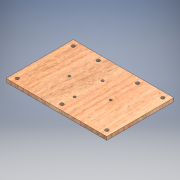
# Autodesk Inventor part: top
Saved by Autodesk Inventor 2018 (Build 220112000, 112)
## iProperties
Created: 2019-06-17
Part Number: top
Material: Generic
Document SubType Name: Modeling
Designer: ZEUSLAP
Density: 1 g/cm^3
Appearance: Default
Author: ZEUSLAP
Autodesk Inventor part; units mm, degrees
ref_plane "YZ Plane" through (0, 0, 0) normal (1, 0, 0) x (0, 1, 0)
ref_plane "XZ Plane" through (0, 0, 0) normal (0, 1, 0) x (-1, 0, 0)
ref_plane "XY Plane" through (0, 0, 0) normal (0, 0, 1) x (1, 0, 0)
sketch "Sketch1" plane through (0, 0, 0) normal (0, 0, 1) x (1, 0, 0)
  line L0 (-70, 40) -> (70, 40) construction
  line L1 (70, 40) -> (70, -40) construction
  line L2 (70, -40) -> (-70, -40) construction
  line L3 (-70, -40) -> (-70, 40) construction
  line L4 (90, 60) -> (-90, 60)
  line L5 (-90, 60) -> (-90, -60)
  line L6 (-90, -60) -> (90, -60)
  line L7 (90, -60) -> (90, 60)
  circle A0 centre (-80, -50) radius 3
  circle A1 centre (80, 50) radius 3
  circle A2 centre (0, -50) radius 3
  circle A3 centre (80, -50) radius 3
  circle A4 centre (-80, 50) radius 3
  line L8 (0, 60) -> (0, -60) construction
  line L9 (-90, 0) -> (90, 0) construction
  circle A5 centre (-35, 50) radius 3
  circle A6 centre (35, 50) radius 3
  circle A7 centre (0, 22.5) radius 2.15
  circle A8 centre (0, -27.5) radius 2.15
  circle A9 centre (37, 0) radius 2.15
  circle A10 centre (-37, 0) radius 2.15
  point P0 (0, 0)
  point P1 (-70, 0)
  point P2 (0, 40)
  point P3 (0, 0)
  dimension "d0" = 140
  dimension "d1" = 80
  dimension "d2" = 20
  dimension "d3" = 6
  dimension "d4" = 10
  dimension "d5" = 10
  dimension "d8" = 35
  dimension "d9" = 4.3
  dimension "d10" = 74
  dimension "d11" = 50
  dimension "d12" = 27.5
  constraints: 20 end point, 11 centre point, 8 equal radius, 7 midpoint, 4 parallel, 4 point on line, 2 horizontal alignment, 2 perpendicular, 1 horizontal, 1 vertical alignment, 9 other
  measures "d0" distance of L1.end L2.end
  measures "d1" distance of L0.end L1.end
  measures "d2" distance between parallel lines of L0 L4
  measures "d3" diameter of A4
  measures "d4" distance from line of L5 A4.centre
  measures "d5" distance from line of L4 A4.centre
  measures "d8" distance from line of L8 A5.centre
  measures "d9" diameter of A7
  measures "d10" distance of A9.centre A10.centre
  measures "d11" distance of A8.centre A7.centre
  measures "d12" distance of A8.centre point (0, 0)
extrude "Extrusion1" add sketch "Sketch1" along normal blind 6
body "Solid1"
